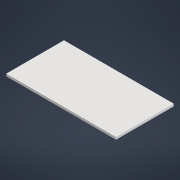
# Autodesk Inventor part: Base
Saved by Autodesk Inventor 2022 (Build 260153000, 153)
## iProperties
Created: 2023-05-09
Part Number: Base
Material: Genérico
Document SubType Name: Modeling
Designer: jpjoa
Density: 1 g/cm^3
Appearance: Padrão
Author: jpjoa
Autodesk Inventor part; units mm, degrees
ref_plane "YZ Plane" through (0, 0, 0) normal (1, 0, 0) x (0, 1, 0)
ref_plane "XZ Plane" through (0, 0, 0) normal (0, 1, 0) x (-1, 0, 0)
ref_plane "XY Plane" through (0, 0, 0) normal (0, 0, 1) x (1, 0, 0)
sketch "Esboço1" plane through (0, 0, 0) normal (0, 1, 0) x (-1, 0, 0)
  line L0 (0, 0) -> (-380, 0)
  line L1 (-380, 0) -> (-380, -95)
  line L2 (-380, -95) -> (0, -95)
  line L3 (0, -95) -> (0, 0)
  point P0 (0, -47.5)
  point P1 (-190, 0)
  dimension "d5" = 380
  dimension "d6" = 95
  constraints: 8 end point, 3 perpendicular, 2 midpoint, 1 horizontal, 1 horizontal alignment, 1 vertical alignment
  measures "d5" distance of L0.start L0.end
  measures "d6" distance of L0.end L1.end
extrude "Extrusão1" add sketch "Esboço1" along normal mid plane 8
equation "\"d5\" = Largura"
equation "\"d6\" = Comprimento"
equation "\"d3\" = Altura"
equation "\"Altura\" = 8"
equation "\"Largura\" = 380"
equation "\"Comprimento\" = 95"
equation "\"Espessura_torre_base\" = 15 * Filamento"
equation "\"Filamento\" = 0.4"
